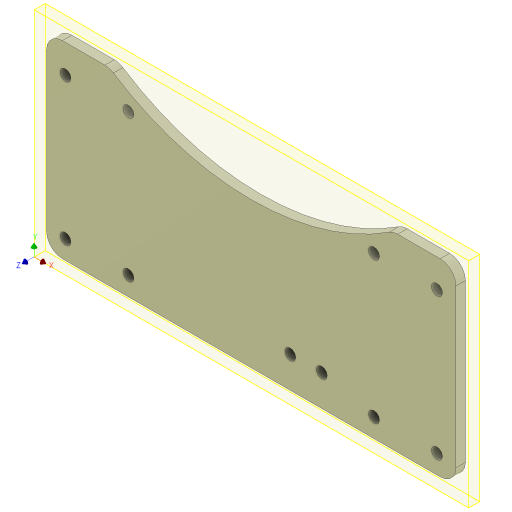
# Autodesk Inventor part: Base plate
Saved by Autodesk Inventor 2024.3 (Build 283343000, 343)
## iProperties
Created: 2025-04-26
Part Number: Base plate
Material: Generic
Document SubType Name: Modeling
Designer: Binara
Density: 1 g/cm^3
Appearance: Default
Author: Binara
Autodesk Inventor part; units mm, degrees
ref_plane "YZ Plane" through (0, 0, 0) normal (1, 0, 0) x (0, 1, 0)
ref_plane "XZ Plane" through (0, 0, 0) normal (0, 1, 0) x (-1, 0, 0)
ref_plane "XY Plane" through (0, 0, 0) normal (0, 0, 1) x (1, 0, 0)
sketch "Sketch1" plane through (0, 0, 0) normal (0, 0, 1) x (1, 0, 0)
  line L0 (-65, -30) -> (65, -30)
  line L1 (65, -30) -> (65, 30)
  line L2 (65, 30) -> (-65, 30)
  line L3 (-65, 30) -> (-65, -30)
  line L4 (-65, -30) -> (65, 30) construction
  line L5 (65, -30) -> (-65, 30) construction
  arc A0 (-45, 30) -> (45, 30) centre (0, 96.6789) ccw
  point P0 (0, 0)
  dimension "d0" = 130
  dimension "d1" = 60
  dimension "d5" = 20
  dimension "d6" = 20
  constraints: 12 end point, 2 midpoint, 2 parallel, 2 point on circle, 2 point on line, 1 centre point, 1 horizontal, 1 perpendicular
  measures "d0" distance of L2.end L1.end
  measures "d1" distance of L1.end L0.end
  measures "d5" distance from line of L1 A0.end
  measures "d6" distance from line of L3 A0.start
extrude "Extrusion1" add sketch "Sketch1" along normal blind 3 contours L3 L2 A0 L1 L0
fillet "Fillet1" radius 5 6 edges at (65, 30, 1.5) (65, -30, 1.5) (-65, -30, 1.5) (-65, 30, 1.5) (45, 30, 1.5) (-45, 30, 1.5)
sketch "Sketch2" plane through (0, 0, 3) normal (0, 0, 1) x (1, 0, 0)
  circle A0 centre (59, -24) radius 1.75
  circle A1 centre (39, -24) radius 1.75
  line L0 (65, -25) -> (65, 25) projected
  line L1 (-60, -30) -> (60, -30) projected
  circle A2 centre (59, 21) radius 1.75
  circle A3 centre (39, 21) radius 1.75
  line L2 (0, -30) -> (0, -45.4947)
  circle A4 centre (-59, -24) radius 1.75
  circle A5 centre (-39, -24) radius 1.75
  line L3 (-65, -25) -> (-65, 25)
  circle A6 centre (-59, 21) radius 1.75
  circle A7 centre (-39, 21) radius 1.75
  point P0 (0, 0)
  dimension "d7" = 3.5
  dimension "d8" = 3.5
  dimension "d9" = 20
  dimension "d10" = 6
  dimension "d11" = 6
  dimension "d14" = 45
  constraints: 8 centre point, 6 symmetric about line, 4 end point, 2 vertical, 1 horizontal alignment, 1 midpoint, 8 other
  measures "d7" diameter of A0
  measures "d8" diameter of A1
  measures "d9" distance of A0.centre A1.centre
  measures "d10" distance from line of L0 A0.centre
  measures "d11" distance from line of L1 A0.centre
  measures "d14" distance of A0.centre A2.centre
extrude "Extrusion2" cut sketch "Sketch2" against normal up to surface (3 mm away)
sketch "Sketch3" plane through (0, 0, 0) normal (0, 0, -1) x (-1, 0, 0)
  circle A0 centre (-12.3926, -20.1) radius 1.75 projected
  circle A1 centre (-22.3926, -20.1) radius 1.75 projected
  point P0 (0, 0)
extrude "Extrusion3" cut sketch "Sketch3" against normal up to surface (3 mm away)
equation "\"d6\" = d5"
body "Solid1"
